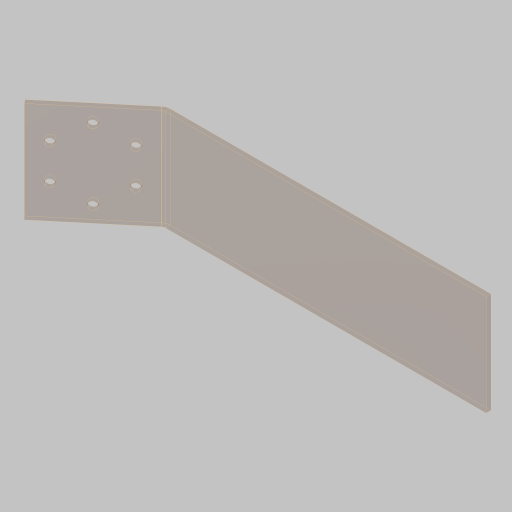
# Autodesk Inventor part: CL7-023
Saved by Autodesk Inventor 2023.5 (Build 275446000, 446)
## iProperties
Created: 2025-04-01
Part Number: CL7-023
Material: Polycarbonate, Smoke
Document SubType Name: Sheet Metal
Designer: slick
Density: 1.2 g/cm^3
Sheet Metal Rule: Default
Appearance: Polycarbonate - Smoked
Author: slick
Autodesk Inventor part; units mm, degrees
ref_plane "YZ Plane" through (0, 0, 0) normal (1, 0, 0) x (0, 1, 0)
ref_plane "XZ Plane" through (0, 0, 0) normal (0, 1, 0) x (-1, 0, 0)
ref_plane "XY Plane" through (0, 0, 0) normal (0, 0, 1) x (1, 0, 0)
sketch "Sketch1" plane through (0, 0, 0) normal (0, 0, 1) x (1, 0, 0)
  line L0 (101.6, -31.75) -> (-101.6, -31.75)
  line L1 (-101.6, -31.75) -> (-101.6, 31.75)
  line L2 (-101.6, 31.75) -> (101.6, 31.75)
  line L3 (101.6, 31.75) -> (101.6, -31.75)
  line L4 (101.6, -31.75) -> (-101.6, 31.75) construction
  line L5 (-101.6, -31.75) -> (101.6, 31.75) construction
  point P0 (0, 0)
  dimension "d0" = 63.5
  dimension "d1" = 203.2
  measures "d0" distance between parallel lines of L2 L0
  measures "d1" distance of L1.end L2.end
extrude "Plate1" add sketch "Sketch1" along normal blind 3.048
sketch "Sketch2" plane through (-101.6, -31.75, 3.048) normal (-0.6427876, 0, -0.7660444) x (0, -1, 0)
  line L0 (-63.5, 0) -> (0, 0)
  line L1 (0, 0) -> (0, 62.3906)
  line L2 (0, 62.3906) -> (-63.5, 62.3906)
  line L3 (-63.5, 62.3906) -> (-63.5, 0)
  constraints: 6 end point, 1 horizontal, 1 perpendicular, 1 vertical
edge flange "Flange1" height 63.5 angle 40 thickness 3.048 bend radius 3.048 thickness toward (-0.6427876, 0, -0.7660444) relief straight relief width 3.048 relief depth 1.524 edges at (-101.6, 0, 3.048) wall of the first edge with corners at (-101.6, 31.75, 3.048) (-101.6, -31.75, 3.048) (-149.394, -31.75, 43.1519) (-149.394, 31.75, 43.1519)
bend "Bend1"
corner "Corner1"
sketch "Sketch3" plane through (-151.3532, -31.75, 40.817) normal (-0.6427876, 0, -0.7660444) x (-0.7660444, 0, 0.6427876)
  circle A0 centre (-30.6406, 31.75) radius 22.225 construction
  line L0 (-61.2812, 63.5) -> (0, 63.5) construction
  point P0 (-142.18, 31.75)
  point P1 (-30.6406, 63.5)
  point P2 (-30.6406, 53.975)
  point P3 (-49.888, 42.8625)
  point P4 (-49.888, 20.6375)
  point P5 (-30.6406, 9.525)
  point P6 (-11.3932, 20.6375)
  point P7 (-11.3932, 42.8625)
  dimension "d13" = 44.45
  dimension "d16" = 360
  constraints: 3 vertical alignment, 1 horizontal alignment, 1 midpoint, 9 other
hole "Hole1" at (-127.8811, 22.225, 21.1216) at (-113.1368, 11.1125, 8.7496) at (-113.1368, -11.1125, 8.7496) at (-127.8811, -22.225, 21.1216) at (-142.6255, -11.1125, 33.4936) at (-142.6255, 11.1125, 33.4936) direction (0.6427876, 0, 0.7660444) diameter 5.1054 depth 3.048 tip angle 118 clearance for "Flat Head Machine Screw (82)" size "#10" standard "Ansi Unified Screw Threads"
equation "\"d23\" = Thickness"
equation "\"d2\" = Thickness"
equation "\"d3\" = BendReliefWidth"
equation "\"d4\" = BendReliefDepth"
equation "\"d5\" = MinimumRemnant"
equation "\"d6\" = TransitionRadius"
equation "\"d9\" = BendRadius"
equation "\"d10\" = CornerReliefSize"
equation "\"d11\" = GapSize"
equation "\"d12\" = JacobiRadiusSize"
equation "\"BendRadius\" = Thickness"
equation "\"BendReliefWidth\" = Thickness"
equation "\"BendReliefDepth\" = 0.5 * Thickness"
equation "\"CornerReliefSize\" = 4 * Thickness"
equation "\"MinimumRemnant\" = 2 * Thickness"
equation "\"TransitionRadius\" = BendRadius"
equation "\"JacobiRadiusSize\" = BendRadius"
equation "\"GapSize\" = Thickness"
equation "\"Thickness\" = 3.048"
body "Solid1"
